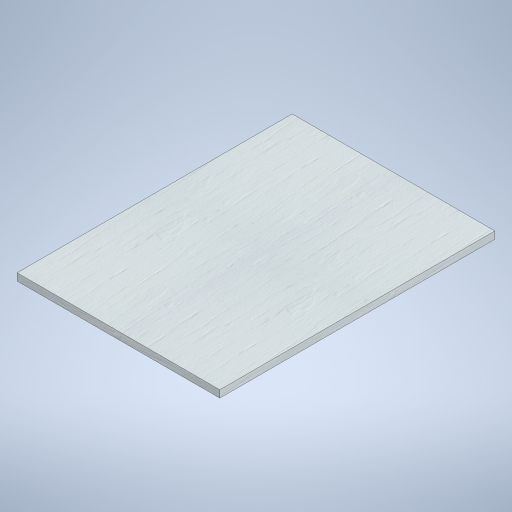
# Autodesk Inventor part: BOTTOM_CETIN_PART_BOX
Saved by Autodesk Inventor 2023 (Build 270158000, 158)
## iProperties
Created: 2024-02-20
Part Number: BOTTOM_CETIN_PART_BOX
Material: PVC, Unplasticized
Document SubType Name: Sheet Metal
Designer: vraco
Density: 1.29 g/cm^3
Sheet Metal Rule: Default_mm
Appearance: Wood - Painted White
Author: vraco
Autodesk Inventor part; units mm, degrees
ref_plane "YZ Plane" through (0, 0, 0) normal (1, 0, 0) x (0, 1, 0)
ref_plane "XZ Plane" through (0, 0, 0) normal (0, 1, 0) x (-1, 0, 0)
ref_plane "XY Plane" through (0, 0, 0) normal (0, 0, 1) x (1, 0, 0)
sketch "Sketch1" plane through (0, 0, 0) normal (0, 1, 0) x (-1, 0, 0)
  line L0 (0, -133) -> (0, 133)
  line L1 (-73, 0) -> (123, 0)
  line L2 (95, 95) -> (-45, 95)
  line L3 (-45, 95) -> (-45, -95)
  line L4 (-45, -95) -> (95, -95)
  line L5 (95, -95) -> (95, 95)
  point P0 (0, 0)
  dimension "d0" = 190
  dimension "d1" = 140
  dimension "d2" = 95
  measures "d0" distance of L2.end L3.end
  measures "d1" distance of L3.end L4.end
  measures "d2" distance between parallel lines of L0 L5
extrude "Plate1" add sketch "Sketch1" along normal blind 5
equation "\"d3\" = Thickness"
equation "\"BendRadius\" = Thickness"
equation "\"BendReliefWidth\" = Thickness"
equation "\"BendReliefDepth\" = 0.5 * Thickness"
equation "\"TransitionRadius\" = BendRadius"
equation "\"JacobiRadiusSize\" = BendRadius"
equation "\"GapSize\" = Thickness"
equation "\"Thickness\" = 5"
body "Solid1"
